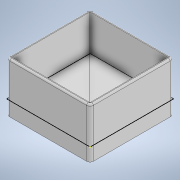
# Autodesk Inventor part: TubeExpander2
Saved by Autodesk Inventor 2020 (Build 240168000, 168)
## iProperties
Created: 2020-04-24
Part Number: TubeExpander2
Material: Типовые
Document SubType Name: Modeling
Designer: Михаил
Density: 1 g/cm^3
Appearance: По умолчанию
Author: Михаил
Autodesk Inventor part; units mm, degrees
sketch "Эскиз1" plane through (0, 0, 0) normal (0, 1, 0) x (-1, 0, 0)
  line L0 (0, 0) -> (50, 0)
  line L1 (50, 0) -> (50, -50)
  line L2 (50, -50) -> (0, -50)
  line L3 (0, -50) -> (0, 0)
  dimension "d0" = 50
  dimension "d1" = 50
  constraints: 8 end point, 2 parallel, 1 horizontal, 1 perpendicular
  measures "d0" distance of L1.end L2.end
  measures "d1" distance of L0.end L1.end
extrude "Выдавливание1" add sketch "Эскиз1" along normal blind 30
sketch "Эскиз2" plane through (0, 30, 0) normal (0, 1, 0) x (1, 0, 0)
  line L0 (-48.5, 1.5) -> (-1.5, 1.5)
  line L1 (-1.5, 1.5) -> (-1.5, 48.5)
  line L2 (-1.5, 48.5) -> (-48.5, 48.5)
  line L3 (-48.5, 48.5) -> (-48.5, 1.5)
  line L4 (-50, 0) -> (0, 0) projected
  line L5 (-50, 50) -> (-50, 0) projected
  dimension "d4" = 47
  dimension "d5" = 47
  dimension "d6" = 1.5
  dimension "d7" = 1.5
  constraints: 8 end point, 2 parallel, 1 horizontal, 1 perpendicular
  measures "d4" distance of L2.end L1.end
  measures "d5" distance of L1.end L0.end
  measures "d6" distance between parallel lines of L4 L0
  measures "d7" distance between parallel lines of L5 L3
extrude "Выдавливание2" cut sketch "Эскиз2" against normal blind 28.5
ref_plane "РабПлоскость2" through (0, 8.5, 0) normal (0, 1, 0) x (1, 0, 0)
sketch "Эскиз9" plane through (0, 8.5, 0) normal (0, 1, 0) x (1, 0, 0)
  line L0 (-1.5, 1.5) -> (-48.5, 1.5) projected
  line L1 (-48.5, 48.5) -> (-1.5, 48.5) projected
  line L2 (-1.5, 1.5) -> (-48.5, 1.5)
  line L3 (-48.5, 1.5) -> (-48.5, 48.5)
  line L4 (-48.5, 48.5) -> (-1.5, 48.5)
  line L5 (-1.5, 48.5) -> (-1.5, 1.5)
  line L6 (-50, 0) -> (0, 0) projected
  line L7 (0, 0) -> (0, 50) projected
  line L8 (-50, 0) -> (0, 0)
  line L9 (0, 0) -> (0, 50)
  line L10 (0, 50) -> (-50, 50)
  line L11 (-50, 50) -> (-50, 0)
  constraints: 16 end point, 4 parallel, 2 horizontal, 2 perpendicular
ref_plane "РабПлоскость3" through (-48.5, 8.5, -48.5) normal (0, -0.9891, -0.1473) x (1, 0, 0)
sketch "Эскиз11" plane through (-48.5, 8.5, -48.5) normal (0, -0.9891, -0.1473) x (1, 0, 0)
  line L0 (0, -3.1672) -> (0, 1.0312) projected
  line L1 (47, 47.5184) -> (0, 47.5184) projected
  line L2 (0, 0.0492) -> (47, 0.0492)
  line L3 (47, 0.0492) -> (47, 47.5184)
  line L4 (47, 47.5184) -> (0, 47.5184)
  line L5 (0, 47.5184) -> (0, 0.0492)
  point P0 (48.5, 49.223)
  constraints: 8 end point, 2 parallel, 1 horizontal, 1 perpendicular, 1 point on line
extrude "Выдавливание6" add sketch "Эскиз11" along normal blind 5
ref_plane "РабПлоскость4" through (0, 0, 0) normal (0, -1, 0) x (1, 0, 0)
split "Разделение1" plane through (0, 0, 0) removes the side toward (0, -1, 0)
ref_plane "РабПлоскость6" through (-48.5, 8.5, -1.5) normal (-0.1473, -0.9891, 0) x (0, 0, -1)
sketch "Эскиз12" plane through (-48.5, 8.5, -1.5) normal (-0.1473, -0.9891, 0) x (0, 0, -1)
  line L0 (47, 43.32) -> (47, 47.5184) projected
  line L1 (0, 0.2532) -> (47, 0.2532)
  line L2 (47, 0.2532) -> (47, 47.5184)
  line L3 (47, 47.5184) -> (0, 47.5184)
  line L4 (0, 47.5184) -> (0, 0.2532)
  point P0 (-1.5, 49.223)
  constraints: 8 end point, 2 parallel, 1 horizontal, 1 perpendicular
extrude "Выдавливание7" add sketch "Эскиз12" along normal blind 50
split "Разделение2" plane through (0, 0, 0) removes the side toward (0, -1, 0)
sketch "Эскиз13" plane through (0, 0, 0) normal (0, -1, 0) x (1, 0, 0)
  circle A0 centre (-10, -10) radius 2.45
  line L0 (-50, 0) -> (0, 0) projected
  line L1 (0, 0) -> (0, -50) projected
  dimension "d33" = 4.9
  dimension "d34" = 10
  dimension "d35" = 10
  constraints: 1 centre point
  measures "d33" diameter of A0
  measures "d34" distance from line of L0 A0.centre
  measures "d35" distance from line of A0.centre L1
extrude "Выдавливание8" add sketch "Эскиз13" along normal blind 4
sketch "Эскиз14" plane through (-10, -4, -10) normal (0, -1, 0) x (1, 0, 0)
  circle A0 centre (0, 0) radius 2
  point P0 (10, 10)
  dimension "d38" = 4
  constraints: 1 centre point
  measures "d38" diameter of A0
extrude "Выдавливание9" cut sketch "Эскиз14" against normal blind 40
fillet "Сопряжение2" radius 2 4 edges at (0, 15, 0) (0, 15, -50) (-50, 15, -50) (-50, 15, 0)
fillet "Сопряжение3" radius 1 8 edges at (-0.5858, 30, -49.4142) (-25, 30, -50) (-49.4142, 30, -49.4142) (-50, 30, -25) (-49.4142, 30, -0.5858) (-25, 30, 0) (-0.5858, 30, -0.5858) (0, 30, -25)
sketch "Эскиз15" plane through (0, 8.5, 0) normal (0, 1, 0) x (1, 0, 0)
  point P0 (0, 0)
